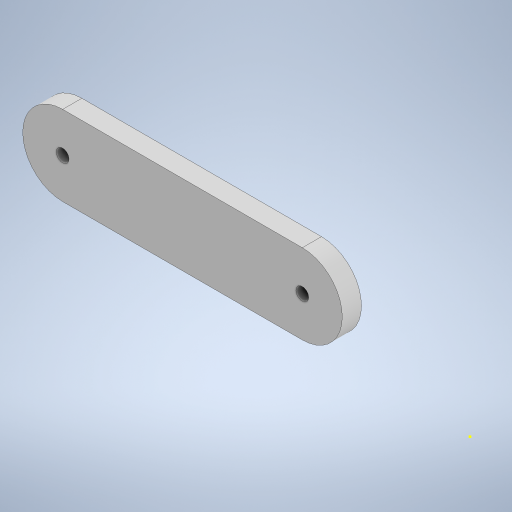
# Autodesk Inventor part: Large Rod
Saved by Autodesk Inventor 2024 (Build 280153000, 153)
## iProperties
Created: 2024-03-08
Part Number: Large Rod
Material: Generic
Document SubType Name: Modeling
Designer: ddcos
Density: 1 g/cm^3
Appearance: Default
Author: ddcos
Autodesk Inventor part; units mm, degrees
ref_plane "YZ Plane" through (0, 0, 0) normal (1, 0, 0) x (0, 1, 0)
ref_plane "XZ Plane" through (0, 0, 0) normal (0, 1, 0) x (-1, 0, 0)
ref_plane "XY Plane" through (0, 0, 0) normal (0, 0, 1) x (1, 0, 0)
sketch "Sketch1" plane through (0, 0, 0) normal (0, 0, 1) x (1, 0, 0)
  line L0 (0, 0) -> (-140, 0)
  line L1 (-140, 0) -> (-140, 25)
  line L2 (-140, 25) -> (0, 25)
  line L3 (0, 25) -> (0, 0)
  dimension "d0" = 140
  dimension "d1" = 25
  constraints: 8 end point, 2 parallel, 1 horizontal, 1 perpendicular
  measures "d0" distance of L1.end L2.end
  measures "d1" distance of L2.end L0.start
extrude "Extrusion1" add sketch "Sketch1" along normal blind 25
sketch "Sketch4" plane through (0, 0, 25) normal (0, 0, 1) x (1, 0, 0)
  point P0 (0, 0)
sketch "Sketch5" plane through (0, 0, 25) normal (0, 0, 1) x (1, 0, 0)
  line L0 (0, 25) -> (-140, 25) projected
  line L1 (0, 0) -> (-40, 0)
  line L2 (-40, 0) -> (-40, 25)
  line L3 (-40, 25) -> (0, 25)
  line L4 (0, 25) -> (0, 0)
  dimension "d16" = 40
  constraints: 8 end point, 2 parallel, 1 horizontal, 1 perpendicular, 1 point on line
  measures "d16" distance of L2.end L3.end
extrude "Extrusion4" cut sketch "Sketch5" against normal blind 100
sketch "Sketch6" plane through (-40, 0, 25) normal (1, 0, 0) x (0, 0, -1)
  line L0 (25, 25) -> (0, 25) projected
  line L1 (25, 0) -> (6, 0)
  line L2 (6, 0) -> (6, 25)
  line L3 (6, 25) -> (25, 25)
  line L4 (25, 25) -> (25, 0)
  dimension "d19" = 19
  constraints: 8 end point, 2 parallel, 1 horizontal, 1 perpendicular, 1 point on line
  measures "d19" distance of L2.end L3.end
extrude "Extrusion5" cut sketch "Sketch6" against normal blind 100
sketch "Sketch7" plane through (0, 0, 25) normal (0, 0, 1) x (1, 0, 0)
  circle A0 centre (-52.5, 12.5) radius 12.5
  circle A1 centre (-127.5, 12.5) radius 12.5
  line L0 (-40, 0) -> (-40, 25) projected
  line L1 (-140, 0) -> (-40, 0) projected
  line L2 (-140, 25) -> (-140, 0) projected
  circle A2 centre (-127.5, 12.5) radius 2
  circle A3 centre (-52.5, 12.5) radius 2
  line L3 (-40, 25) -> (-140, 25) projected
  point P0 (0, 0)
  point P1 (-52.5, 25)
  point P2 (-40, 12.5)
  point P3 (-52.5, 0)
  point P4 (-127.5, 25)
  point P5 (-140, 12.5)
  point P6 (-127.5, 0)
  dimension "d22" = 25
  dimension "d23" = 25
  dimension "d24" = 12.5
  dimension "d25" = 12.5
  dimension "d26" = 12.5
  dimension "d27" = 12.5
  dimension "d28" = 4
  dimension "d29" = 4
  constraints: 4 centre point, 2 coincident
  measures "d22" diameter of A0
  measures "d23" diameter of A1
  measures "d24" distance from line of L0 A0.centre
  measures "d25" distance from line of L1 A0.centre
  measures "d26" distance from line of L1 A1.centre
  measures "d27" distance from line of L2 A1.centre
  measures "d28" diameter of A2
  measures "d29" diameter of A3
extrude "Extrusion6" cut sketch "Sketch7" against normal blind 100 contours L0 L1 A0 | A0 L3 L0 | A1 L2 L3 | L1 L2 A1 | A2 | A3
body "Solid1"
